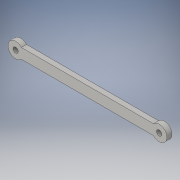
# Autodesk Inventor part: Caufield_Linkage_Arm
Saved by Autodesk Inventor 2016 (Build 200138000, 138)
## iProperties
Created: 2018-01-10
Part Number: Caufield_Linkage_Arm
Material: Generic
Document SubType Name: Modeling
Designer: caufield58738
Density: 1 g/cm^3
Appearance: Default
Mass: 2.01542 g
Surface Area: 19.9973 cm^2
Volume: 2.01542 cm^3
Author: caufield58738
Autodesk Inventor part; units mm, degrees
ref_plane "YZ Plane" through (0, 0, 0) normal (1, 0, 0) x (0, 1, 0)
ref_plane "XZ Plane" through (0, 0, 0) normal (0, 1, 0) x (-1, 0, 0)
ref_plane "XY Plane" through (0, 0, 0) normal (0, 0, 1) x (1, 0, 0)
sketch "Linkage Sketch" plane through (0, 0, 0) normal (0, 0, 1) x (1, 0, 0)
  arc A0 (3.5498, 3.175) -> (3.5498, -3.175) centre (0, 0) ccw
  line L0 (3.5498, 3.175) -> (85.3502, 3.175)
  line L1 (85.3502, 3.175) -> (85.3502, -3.175) construction
  line L2 (85.3502, -3.175) -> (3.5498, -3.175)
  line L3 (3.5498, -3.175) -> (3.5498, 3.175) construction
  arc A1 (85.3502, -3.175) -> (85.3502, 3.175) centre (88.9, 0) ccw
  dimension "d0" = 9.525
  dimension "d1" = 6.35
  dimension "d3" = 9.525
  dimension "d14" = 88.9
  constraints: 8 end point, 4 point on circle, 3 coincident, 2 centre point, 2 parallel, 1 horizontal, 1 perpendicular
  measures "d0" diameter of A0
  measures "d1" distance of L0.end L1.end
  measures "d3" diameter of A1
  measures "d14" distance of A1.centre point (0, 0)
extrude "Linkeage extrution" add sketch "Linkage Sketch" against normal blind 3.175
hole "Linkage holes" at (0, 0, 0) at (88.9, 0, 0) direction (0, 0, -1) diameter 3.2512 end through all
body "Solid1"
